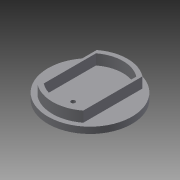
# Autodesk Inventor part: Tapa 3
Saved by Autodesk Inventor 2013 (Build 170138000, 138)
## iProperties
Created: 2014-07-04
Part Number: Tapa 3
Material: Genérico
Document SubType Name: Chapa
Designer: Administrador
Density: 1 g/cm^3
Sheet Metal Rule: Por defecto_mm
Author: Administrador
Autodesk Inventor part; units mm, degrees
ref_plane "YZ Plane" through (0, 0, 0) normal (1, 0, 0) x (0, 1, 0)
ref_plane "XZ Plane" through (0, 0, 0) normal (0, 1, 0) x (-1, 0, 0)
ref_plane "XY Plane" through (0, 0, 0) normal (0, 0, 1) x (1, 0, 0)
sketch "Boceto1" plane through (0, 0, 0) normal (0, 0, 1) x (1, 0, 0)
  line L0 (13, 15.1987) -> (13, -15.1987)
  arc A0 (13, 15.1987) -> (-13, 15.1987) centre (0, 0) ccw
  line L1 (-10.89, 14.1053) -> (-10.89, -14.1053)
  arc A1 (10.89, 14.1053) -> (-10.89, 14.1053) centre (0, 0) ccw
  line L2 (-13, -15.1987) -> (-13, 15.1987)
  arc A2 (-10.89, -14.1053) -> (10.89, -14.1053) centre (0, 0) ccw
  arc A3 (-13, -15.1987) -> (13, -15.1987) centre (0, 0) ccw
  line L3 (10.89, 14.1053) -> (10.89, -14.1053)
  line L4 (-9.6976, 12.5455) -> (-9.6976, -12.3312)
  arc A4 (9.5084, 12.5455) -> (-9.6976, 12.5455) centre (-0.0946, 0.1071) ccw
  arc A5 (-9.6976, -12.3312) -> (9.5084, -12.3312) centre (-0.0946, 0.1071) ccw
  line L5 (9.5084, 12.5455) -> (9.5084, -12.3312)
  constraints: 12 end point, 12 point on circle, 6 centre point
extrude "Extrusión1" add sketch "Boceto1" along normal blind 5 contours A1 L3 A2 L1
sketch "Boceto2" plane through (0, 0, 0) normal (0, 0, -1) x (-1, 0, 0)
  arc A0 (-9.5084, -12.3312) -> (9.6976, -12.3312) centre (0.0946, 0.1071) ccw projected
  arc A1 (-10.89, -14.1053) -> (10.89, -14.1053) centre (0, 0) ccw projected
  arc A2 (13.13, 15.0742) -> (-12.87, 15.0742) centre (0.13, -0.1245) ccw
  arc A3 (-12.87, -15.0742) -> (12.87, -15.0742) centre (0, 0.2347) ccw
  circle A4 centre (0, 0) radius 20
  line L0 (-12.87, -15.0742) -> (-12.87, -12.3254)
  line L1 (-12.87, 12.3254) -> (-12.87, 15.0742)
  line L2 (12.87, 12.3254) -> (13, 9.0726)
  line L3 (12.87, -12.3254) -> (12.87, -15.0742)
  dimension "d2" = 40
  constraints: 9 point on circle, 8 end point, 3 centre point
  measures "d2" diameter of A4
extrude "Extrusión2" add sketch "Boceto2" along normal blind 3
sketch "Boceto3" plane through (0, 0, -3) normal (0, 0, -1) x (-1, 0, 0)
  arc A0 (0.9994, -13.463) -> (-0.9994, -13.463) centre (0, 0) ccw
  arc A1 (-0.9994, -13.463) -> (0.9994, -13.463) centre (0, -13.4987) ccw
  dimension "d5" = 27
  dimension "d6" = 2
  constraints: 4 point on circle, 2 centre point
  measures "d5" diameter of A0
  measures "d6" diameter of A1
extrude "Extrusión3" cut sketch "Boceto3" against normal blind 0.5
hole "Hole1" at (-0.23, -7.8199, -2.5) direction (0, 0, 1) diameter 2 end through all
equation "\"d16\" = Grosor"
equation "\"Radio_pliegue\" = Grosor"
equation "\"Anchura_desahogo_plegado\" = Grosor"
equation "\"Profundidad_desahogo_plegado\" = 0.5 * Grosor"
equation "\"Tamaño_destalonado\" = 4 * Grosor"
equation "\"Remanente_mínimo\" = 2 * Grosor"
equation "\"Radiodetransición\" = Radio_pliegue"
equation "\"Tamaño_de_radio_de_Jacobi\" = Radio_pliegue"
equation "\"TamañoSeparación\" = Grosor"
equation "\"Grosor\" = 0.5"
